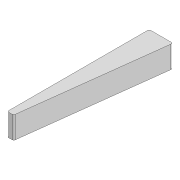
# Autodesk Inventor part: Wedge - V2
Saved by Autodesk Inventor 2020 (Build 240168000, 168)
## iProperties
Created: 2020-08-11
Part Number: Wedge - V2
Material: Generic
Document SubType Name: Modeling
Designer: Dan Wikman
Density: 1 g/cm^3
Appearance: Default
Author: Dan Wikman
Autodesk Inventor part; units mm, degrees
ref_plane "YZ Plane" through (0, 0, 0) normal (1, 0, 0) x (0, 1, 0)
ref_plane "XZ Plane" through (0, 0, 0) normal (0, 1, 0) x (-1, 0, 0)
ref_plane "XY Plane" through (0, 0, 0) normal (0, 0, 1) x (1, 0, 0)
sketch "Sketch1" plane through (0, 0, 0) normal (0, 1, 0) x (-1, 0, 0)
  line L0 (7.1803, 16.0154) -> (7.1803, -27.9846)
  line L1 (6.6803, -28.4846) -> (0.2201, -28.4846)
  line L2 (-0.2762, -27.9236) -> (5.1264, 16.0764)
  line L3 (5.6226, 16.5154) -> (6.6803, 16.5154)
  arc A0 (6.6803, -28.4846) -> (7.1803, -27.9846) centre (6.6803, -27.9846) ccw
  arc A1 (-0.2762, -27.9236) -> (0.2201, -28.4846) centre (0.2201, -27.9846) ccw
  arc A2 (7.1803, 16.0154) -> (6.6803, 16.5154) centre (6.6803, 16.0154) ccw
  arc A3 (5.6226, 16.5154) -> (5.1264, 16.0764) centre (5.6226, 16.0154) ccw
  point P0 (0, 0)
  point P1 (7.1803, 16.5154)
  point P2 (7.1803, -28.4846)
  point P3 (5.1803, 16.5154)
  dimension "d0" = 45
  dimension "d1" = 7
  dimension "d2" = 2
  dimension "d3" = 0.5
  dimension "d4" = 0.5
  dimension "d5" = 0.5
  constraints: 8 end point, 8 point on circle, 8 tangent, 6 point on line, 4 centre point, 1 equal radius, 1 parallel, 1 perpendicular, 1 vertical
  measures "d0" distance of point (7.18, 16.515) point (7.18, -28.485)
  measures "d1" angle of L0 L2
  measures "d2" distance of point (5.18, 16.515) point (7.18, 16.515)
  measures "d3" radius of A0
  measures "d4" radius of A1
  measures "d5" radius of A2
extrude "Extrusion1" add sketch "Sketch1" along normal blind 7
body "Solid1"
